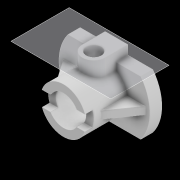
# Autodesk Inventor part: 4-刘宇昂-20202261064
Saved by Autodesk Inventor 2020 (Build 240168000, 168)
## iProperties
Created: 2020-10-16
Part Number: 4-刘宇昂-20202261064
Material: 常规
Document SubType Name: Modeling
Designer: NH55
Density: 1 g/cm^3
Appearance: 默认
Author: NH55
Autodesk Inventor part; units mm, degrees
ref_plane "YZ Plane" through (0, 0, 0) normal (1, 0, 0) x (0, 1, 0)
ref_plane "XY Plane" through (0, 0, 0) normal (0, 0, 1) x (1, 0, 0)
sketch "草图1" plane through (0, 0, 0) normal (0, 0, 1) x (1, 0, 0)
  line L0 (-24, 18) -> (24, 18)
  line L1 (24, -18) -> (-24, -18)
  arc A0 (24, -18) -> (24, 18) centre (0, 0) ccw
  arc A1 (-24, 18) -> (-24, -18) centre (0, 0) ccw
  circle A2 centre (0, 0) radius 10
  circle A3 centre (0, 0) radius 15
  point P0 (0, 18)
  point P1 (0, -18)
  point P2 (30, 0)
  point P3 (-30, 0)
  dimension "d0" = 30
  dimension "d1" = 36
  dimension "d2" = 20
  dimension "d3" = 30
  constraints: 6 point on circle, 4 centre point, 4 end point, 3 coincident, 2 horizontal alignment, 2 midpoint, 2 parallel, 2 vertical alignment, 1 concentric, 1 horizontal
  measures "d0" radius of A0
  measures "d1" distance between parallel lines of L1 L0
  measures "d2" diameter of A2
  measures "d3" diameter of A3
extrude "拉伸1" add sketch "草图1" along normal blind 8 contours L0 A0 L1 A1
extrude "拉伸2" add sketch "草图1" along normal blind 35 contours A3
sketch "草图2" plane through (0, 0, 0) normal (1, 0, 0) x (0, 1, 0)
  point P0 (0, 0)
ref_plane "工作平面1" through (0, 24, 0) normal (0, 1, 0) x (-1, 0, 0)
sketch "草图3" plane through (0, 24, 0) normal (0, 1, 0) x (-1, 0, 0)
  line L0 (-24, 0) -> (24, 0) projected
  line L1 (24, 0) -> (24, 8) projected
  line L2 (-24, 8) -> (24, 8) projected
  line L3 (-24, 0) -> (-24, 8) projected
  line L4 (15, 35) -> (-15, 35) projected
  line L5 (-15, 8) -> (15, 8) projected
  line L6 (24, 0) -> (24, 0) projected
  line L7 (24, 0) -> (24, 8) projected
  line L8 (24, 8) -> (24, 8) projected
  line L9 (24, 0) -> (24, 8) projected
  line L10 (-24, 0) -> (-24, 0) projected
  line L11 (-24, 0) -> (-24, 8) projected
  line L12 (-24, 8) -> (-24, 8) projected
  line L13 (-24, 0) -> (-24, 8) projected
  line L14 (24, 0) -> (-24, 0) projected
  line L15 (-7.5, 0) -> (-7.5, 15)
  arc A0 (7.5, 15) -> (-7.5, 15) centre (0, 15) ccw
  line L16 (7.5, 15) -> (7.5, 0)
  point P0 (0, 0)
  point P1 (0, 22.5)
  point P2 (0, 0)
  point P3 (0, 0)
  point P4 (7.5, 0)
  dimension "d9" = 7.5
  dimension "d10" = 15
  constraints: 4 end point, 3 point on circle, 3 vertical alignment, 2 tangent, 2 vertical, 1 centre point, 1 midpoint, 4 other
  measures "d9" radius of A0
  measures "d10" distance of L16.start L16.end
extrude "拉伸3" add sketch "草图3" against normal up to surface contours L15 L2 L16 L0 | L15 A0 L16 L2 round surface about axis through (0, 0, 0) along (0, 0, 1) radius 15 far side no
sketch "草图4" plane through (0, 24, 0) normal (0, 1, 0) x (1, 0, 0)
  line L0 (-7.5, 0) -> (-7.5, -15) projected
  arc A0 (-7.5, -15) -> (7.5, -15) centre (0, -15) ccw projected
  line L1 (7.5, -15) -> (7.5, 0) projected
  line L2 (7.5, 0) -> (-7.5, 0) projected
  circle A1 centre (0, -15) radius 5
  point P0 (0, 0)
  dimension "d13" = 10
  constraints: 1 centre point, 1 coincident
  measures "d13" diameter of A1
extrude "拉伸4" cut sketch "草图4" against normal up to surface contours A1 round surface about axis through (0, 0, 0) along (0, 0, 1) radius 10 far side no
sketch "草图5" plane through (0, 0, 35) normal (0, 0, 1) x (1, 0, 0)
  line L0 (-15, -5.1442) -> (15, -5.1442)
  line L1 (15, -5.1442) -> (15, 4.8558)
  line L2 (15, 4.8558) -> (-15, 4.8558)
  line L3 (-15, 4.8558) -> (-15, -5.1442)
  circle A0 centre (0, 0) radius 15 projected
  circle A1 centre (0, 0) radius 10 projected
  circle A2 centre (0, 0) radius 15 projected
  point P0 (0, -5.1442)
  point P1 (0, 4.8558)
  point P2 (-14.1923, 4.8558)
  point P3 (-14.0903, -5.1442)
  point P4 (14.0903, -5.1442)
  point P5 (14.1923, 4.8558)
  dimension "d16" = 10
  constraints: 8 end point, 2 midpoint, 2 parallel, 2 tangent, 2 vertical alignment, 1 horizontal, 1 perpendicular
  measures "d16" distance of L2.end L0.start
extrude "拉伸5" cut sketch "草图5" against normal blind 5 contours A0 L2 A1 L0 | A1 L2 L0 | L0 A1 L2 A0
sketch "草图6" plane through (0, 0, 0) normal (0, 1, 0) x (-1, 0, 0)
  line L0 (24, 8) -> (-24, 8) projected
  line L1 (-27, 8) -> (-15, 25.1378)
  line L2 (-15, 8) -> (-15, 30) projected
  circle A0 centre (0, 15) radius 5 projected
  line L3 (7.5, 0) -> (7.5, 15) projected
  arc A1 (7.5, 15) -> (-7.5, 15) centre (0, 15) ccw projected
  line L4 (-7.5, 15) -> (-7.5, 0) projected
  line L5 (-7.5, 0) -> (7.5, 0) projected
  line L6 (-7.5, 0) -> (7.5, 0) projected
  line L7 (-24, 8) -> (-30, 8) projected
  point P0 (0, 0)
  dimension "d21" = 55
  dimension "d22" = 27
  constraints: 2 end point, 1 midpoint, 1 point on line
  measures "d21" angle of L0 L1
  measures "d22" horizontal distance of point (0, 0) L1.start
extrude "加强筋1" add sketch "草图6" along normal mid plane 5 rib yes fills toward (-20.959, 16.5402) open curves L1
mirror "镜像1" about plane through (0, 0, 0) normal (1, 0, 0) of "加强筋1"
equation "\"d22\" = 0.5 * d20"
equation "\"d20\" = 54"
